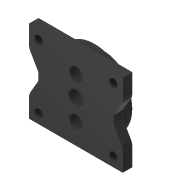
# Autodesk Inventor part: Cap Top Cap
Saved by Autodesk Inventor 2017 (Build 210142000, 142)
## iProperties
Created: 2016-08-05
Part Number: Cap Top Cap
Material: Generic
Document SubType Name: Modeling
Designer: ge937963
Density: 1 g/cm^3
Appearance: Smooth - Black
Mass: 2.34883 g
Surface Area: 15.0001 cm^2
Volume: 2.34883 cm^3
Author: ge937963
Autodesk Inventor part; units mm, degrees
ref_plane "YZ Plane" through (0, 0, 0) normal (1, 0, 0) x (0, 1, 0)
ref_plane "Work Plane1" through (0, 0, 0) normal (0, 0, 1) x (1, 0, 0)
sketch "Sketch1" plane through (0, 0, 0) normal (0, 0, 1) x (1, 0, 0)
  circle A0 centre (0, 0) radius 9.525 projected
  circle A1 centre (0, 0) radius 12.7 projected
  point P0 (0, 0)
extrude "Extrusion1" add sketch "Sketch1" along normal blind 3.175 contours A0 | A1
sketch "Sketch2" plane through (0, 0, 0) normal (0, 0, -1) x (-1, 0, 0)
  circle A0 centre (0, 0) radius 9.025
  point P0 (0, 0)
  dimension "d2" = 18.05
  constraints: 1 centre point, 1 coincident
  measures "d2" diameter of A0
extrude "Extrusion2" add sketch "Sketch2" along normal blind 3.175
sketch "Sketch3" plane through (0, 0, 3.175) normal (0, 0, 1) x (1, 0, 0)
  circle A0 centre (0, 0) radius 2.54
  point P0 (0, 0)
  dimension "d5" = 5.08
  constraints: 1 centre point, 1 coincident
  measures "d5" diameter of A0
extrude "Extrusion3" cut sketch "Sketch3" against normal through all
sketch "Sketch4" plane through (0, 0, 0) normal (0, 1, 0) x (-1, 0, 0)
  line L0 (12.7, 3.175) -> (-12.7, 3.175) projected
  line L1 (-12.7, 3.175) -> (12.7, 3.175)
  line L2 (12.7, 3.175) -> (12.7, 6.35)
  line L3 (12.7, 6.35) -> (-12.7, 6.35)
  line L4 (-12.7, 6.35) -> (-12.7, 3.175)
  point P0 (0, 0)
  dimension "d8" = 3.175
  constraints: 8 end point, 2 parallel, 1 horizontal, 1 perpendicular
  measures "d8" distance of L1.end L2.end
ref_plane "Work Plane2" through (-27.0849, -13.97, -71.335) normal (0, 1, 0) x (0, 0, 1)
extrude "Extrusion4" add sketch "Sketch4" against normal up to surface (13.97 mm away)
sketch "Sketch5" plane through (0, 0, 3.175) normal (0, 0, 1) x (1, 0, 0)
  line L0 (-12.7, 0) -> (-2.54, 0) projected
  arc A0 (2.54, 0) -> (-2.54, 0) centre (0, 0) ccw projected
  line L1 (2.54, 0) -> (12.7, 0) projected
  arc A1 (12.7, 0) -> (-12.7, 0) centre (0, 0) ccw projected
  point P0 (0, 0)
extrude "Extrusion5" add sketch "Sketch5" along normal blind 3.175
sketch "Sketch6" plane through (0, 0, 6.35) normal (0, 0, 1) x (1, 0, 0)
  circle A0 centre (0, 0) radius 1.905
  point P0 (0, 0)
  constraints: 1 centre point, 1 coincident
extrude "Extrusion6" cut sketch "Sketch6" against normal blind 3.175
sketch "Sketch8" plane through (0, 0, 3.175) normal (0, 0, -1) x (-1, 0, 0)
  line L0 (-29.0812, -13.97) -> (27.0849, -13.97) projected
  arc A0 (-1.905, 0) -> (1.905, 0) centre (0, 0) ccw projected
  arc A1 (12.7, 0) -> (-12.7, 0) centre (0, 0) ccw projected
  line L1 (12.7, 0) -> (12.7, -13.97) projected
  line L2 (-12.7, -13.97) -> (12.7, -13.97) projected
  line L3 (-12.7, 0) -> (-12.7, -13.97) projected
  line L4 (15.875, -13.97) -> (15.875, -7.62)
  line L5 (15.4496, -6.0325) -> (12.7, -1.27)
  line L6 (12.7, 0) -> (12.7, -13.97) projected
  arc A2 (15.875, -7.62) -> (15.4496, -6.0325) centre (12.7, -7.62) ccw
  line L7 (-15.875, -13.97) -> (-15.875, -7.62)
  line L8 (-15.4496, -6.0325) -> (-12.7, -1.27)
  line L9 (-12.7, 0) -> (-12.7, -13.97) projected
  arc A3 (-15.4496, -6.0325) -> (-15.875, -7.62) centre (-12.7, -7.62) ccw
  line L10 (2.54, 0) -> (1.905, 0) projected
  arc A4 (2.54, 0) -> (-2.54, 0) centre (0, 0) ccw projected
  line L11 (-1.905, 0) -> (-2.54, 0) projected
  point P0 (0, 0)
  dimension "d21" = 3.175
  dimension "d22" = 3.175
  dimension "d23" = 6.35
  dimension "d24" = 3.175
  dimension "d25" = 3.175
  dimension "d26" = 6.35
  constraints: 8 end point, 4 point on circle, 4 point on line, 4 tangent, 2 centre point, 2 horizontal alignment, 2 vertical
  measures "d21" radius of A2
  measures "d22" distance between parallel lines of L1 L4
  measures "d23" vertical distance of L4.end L5.end
  measures "d24" radius of A3
  measures "d25" distance between parallel lines of L7 L3
  measures "d26" distance from line of L0 A2.centre
extrude "Extrusion8" add sketch "Sketch8" against normal blind 3.175 contours L7 A3 L8 L3 L0 | L1 L5 A2 L4 L0
sketch "Sketch9" plane through (0, 0, 3.175) normal (0, 0, -1) x (-1, 0, 0)
  circle A0 centre (12.7, -10.795) radius 1.397
  circle A1 centre (-12.7, -10.795) radius 1.397
  line L0 (15.875, -13.97) -> (15.875, -7.62) projected
  line L1 (-15.875, -13.97) -> (15.875, -13.97) projected
  line L2 (-15.875, -7.62) -> (-15.875, -13.97) projected
  point P0 (0, 0)
  dimension "d29" = 3.175
  dimension "d30" = 3.175
  dimension "d31" = 2.794
  dimension "d32" = 3.175
  dimension "d33" = 3.175
  constraints: 2 centre point, 1 equal radius
  measures "d29" distance from line of L0 A0.centre
  measures "d30" distance from line of L1 A0.centre
  measures "d31" diameter of A0
  measures "d32" distance from line of L1 A1.centre
  measures "d33" distance from line of L2 A1.centre
extrude "Extrusion9" cut sketch "Sketch9" against normal blind 3.175
sketch "Sketch10" plane through (0, 0, 6.35) normal (0, 0, 1) x (1, 0, 0)
  circle A0 centre (0, 0) radius 2.54
  circle A1 centre (0, 6.985) radius 2.286
  circle A2 centre (0, -6.985) radius 2.286
  circle A3 centre (0, 0) radius 9.025 projected
  dimension "d36" = 5.08
  dimension "d37" = 4.572
  dimension "d38" = 4.572
  dimension "d39" = 6.985
  dimension "d40" = 6.985
  constraints: 3 centre point, 2 vertical alignment, 1 coincident
  measures "d36" diameter of A0
  measures "d37" diameter of A1
  measures "d38" diameter of A2
  measures "d39" distance of A3.centre A2.centre
  measures "d40" distance of point (0, 0) A1.centre
extrude "Extrusion10" cut sketch "Sketch10" against normal through all contours A0
extrude "Extrusion11" cut sketch "Sketch10" against normal blind 5.5563 contours A1 A3 | A3 A1 | A3 A2 | A2 A3
sketch "Sketch11" plane through (0, 0, -3.175) normal (0, 0, -1) x (-1, 0, 0)
  circle A0 centre (0, -6.985) radius 2.286 projected
  circle A1 centre (0, 6.985) radius 2.286 projected
  circle A2 centre (0, -6.985) radius 1.27
  circle A3 centre (0, 6.985) radius 1.27
  point P0 (0, 0)
  dimension "d45" = 2.54
  constraints: 2 centre point, 2 coincident, 1 equal radius
  measures "d45" diameter of A2
extrude "Extrusion12" cut sketch "Sketch11" against normal through all contours A2 | A3
mirror "Mirror1" about plane through (0, 0, 0) normal (0, 1, 0) of "Extrusion8", "Extrusion9", "Extrusion4", "Extrusion11", "Extrusion3", "Extrusion10"
sketch "Sketch12" plane through (-15.875, -13.97, 6.35) normal (0, 0, 1) x (1, 0, 0)
  circle A0 centre (15.875, 13.97) radius 2.2303
  constraints: 1 centre point, 1 coincident
extrude "Extrusion13" cut sketch "Sketch12" against normal blind 25.4
body "Solid1"
